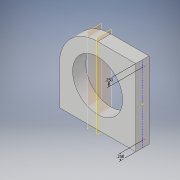
# Autodesk Inventor part: gripperBracket
Saved by Autodesk Inventor 2018.2 (Build 222227000, 227)
## iProperties
Created: 2018-02-13
Part Number: gripperBracket
Material: Generic
Document SubType Name: Modeling
Designer: steele
Density: 1 g/cm^3
Appearance: Default
Author: steele
Autodesk Inventor part; units mm, degrees
ref_plane "XZ Plane" through (0, 0, 0) normal (0, 1, 0) x (-1, 0, 0)
ref_plane "XY Plane" through (0, 0, 0) normal (0, 0, 1) x (1, 0, 0)
sketch "Sketch1" plane through (0, 0, 0) normal (0, 0, 1) x (1, 0, 0)
  circle A0 centre (0, 0) radius 24.13
  arc A1 (0, 36.83) -> (-36.83, 0) centre (0, 0) ccw
  line L0 (0, -36.83) -> (-36.83, -36.83)
  line L1 (-36.83, 0) -> (-36.83, -36.83)
  line L2 (0, 36.83) -> (36.83, 36.83)
  line L3 (0, -36.83) -> (36.83, -36.83)
  line L4 (36.83, 0) -> (36.83, -36.83)
  line L5 (36.83, 0) -> (36.83, 36.83)
  dimension "d0" = 48.26
  dimension "d1" = 73.66
  constraints: 12 end point, 5 tangent, 3 horizontal, 3 perpendicular, 2 centre point, 2 coincident, 2 point on circle
  measures "d0" diameter of A0
  measures "d1" diameter of A1
extrude "Extrusion1" add sketch "Sketch1" along normal mid plane 12.7
sketch "Sketch2" plane through (-36.83, -36.83, 6.35) normal (-1, 0, 0) x (0, 0, 1)
  line L0 (0, 0) -> (-12.7, 0) construction
  line L1 (-6.35, 0) -> (-6.35, 36.83) construction
  point P0 (-6.35, 10.16)
  dimension "d4" = 10.16
  constraints: 2 end point, 1 midpoint, 1 point on line, 1 vertical
  measures "d4" distance from line of point (-6.35, 10.16) L0
hole "Hole1" at (-36.83, -26.67, 0) direction (1, 0, 0) diameter 4.9784 depth 31.75 tip angle 118 thread size "1/4-20 UNC" class "2B" standard "ANSI Unified Screw Threads"
ref_plane "Work Plane1" through (-9.525, 0, 0) normal (1, 0, 0) x (0, 1, 0)
sketch "Sketch3" plane through (36.83, -36.83, 6.35) normal (1, 0, 0) x (0, 0, -1)
  line L0 (0, 73.66) -> (12.7, 73.66) construction
  line L1 (6.35, 73.66) -> (6.35, 0) construction
  line L2 (0, 0) -> (12.7, 0) construction
  point P0 (6.35, 36.83)
  point P1 (6.35, 67.31)
  point P2 (6.35, 6.35)
  dimension "d13" = 6.35
  dimension "d14" = 6.35
  constraints: 2 end point, 2 midpoint, 2 point on line
  measures "d13" distance from line of point (6.35, 67.31) L0
  measures "d14" distance from line of point (6.35, 6.35) L2
equation "\"d0\" = pipeDiameter"
equation "\"d1\" = pipeDiameter + 2 * outerRadius"
equation "\"pipeDiameter\" = 48.26"
equation "\"outerRadius\" = 12.7"
body "Solid1"
